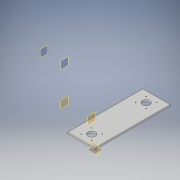
# Autodesk Inventor part: BT001_trajan20_21
Saved by Autodesk Inventor 2022.2 (Build 262287000, 287)
## iProperties
Company: HTBLA Kaindorf
RuleStatus: InUse
Created: 2022-06-05
Part Number: BT001_trajan20_21
Project: Zeichenmaschine_v2
Material: Generisch
Description: Gerüst
Document SubType Name: Modeling
Designer: trajan20
Density: 1 g/cm^3
Appearance: Vorgabe
Mass: 84.0087 g
Surface Area: 376.036 cm^2
Volume: 84.0087 cm^3
AfterDocNew0: iProperties-Editor_aufrufen
Author: jan
Keywords: 2021
Autodesk Inventor part; units mm, degrees
ref_plane "YZ Plane" through (0, 0, 0) normal (1, 0, 0) x (0, 1, 0)
ref_plane "XZ Plane" through (0, 0, 0) normal (0, 1, 0) x (-1, 0, 0)
ref_plane "XY Plane" through (0, 0, 0) normal (0, 0, 1) x (1, 0, 0)
derived "MS000_trajan20_21_Zeichenmaschine_Inventor_Masterskizze.ipt"
sketch "Skizze16" plane through (110, 40, -80) normal (1, 0, 0) x (0, 1, 0)
  line L0 (0, 0) -> (-80, 0)
  line L1 (-80, 0) -> (-80, -5)
  line L2 (-80, -5) -> (0, -5)
  line L3 (0, -5) -> (0, 0)
  point P0 (-40, 80)
sketch "Skizze17" plane through (110, 40, -85) normal (0, 0, -1) x (-1, 0, 0)
  line L0 (110, -322) -> (110, 182)
  line L1 (134, -40) -> (-34, -40)
  point P0 (110, -40)
  point P1 (30, -40)
  point P2 (14.5, -55.5)
  point P3 (45.5, -55.5)
  point P4 (14.5, -24.5)
  point P5 (45.5, -24.5)
extrude "Extrusion3" add sketch "Skizze16" against normal blind 110
sketch "Skizze5" plane through (110, -40, -85) normal (0, 0, -1) x (-1, 0, 0)
  point P0 (110, 40)
  point P1 (30, 40)
  point P2 (30, 40)
  constraints: 1 coincident
hole "Bohrung1" at (95.5, -15.5, -85) at (95.5, 15.5, -85) at (64.5, 15.5, -85) at (64.5, -15.5, -85) direction (0, 0, 1) diameter 2.459 end through all thread size "M3x0.5" class "6H" standard "ISO Metric profile"
hole "Bohrung2" at (80, 0, -85) direction (0, 0, 1) diameter 22 end through all
mirror "Spiegeln1" about plane through (0, 0, -82.5) normal (-1, 0, 0)
ref_plane "Arbeitsebene7" through (120, 40, 0) normal (0, 1, 0) x (-1, 0, 0)
ref_plane "Arbeitsebene8" through (120, -40, 0) normal (0, 1, 0) x (-1, 0, 0)
ref_plane "Arbeitsebene9" through (20, -200, 0) normal (0, -1, 0) x (1, 0, 0)
ref_plane "Arbeitsebene10" through (20, -140, 0) normal (0, -1, 0) x (1, 0, 0)
ref_plane "Arbeitsebene12" through (110, 40, -80) normal (1, 0, 0) x (0, 1, 0)
ref_plane "Arbeitsebene13" through (110, 40, -85) normal (0, 0, -1) x (-1, 0, 0)
equation "\"d5\" = 0.5 * Bas_Haupt_Länge"
equation "\"d14\" = SM_Scheibe_Durchmesser"
equation "\"Bas_Haupt_Länge\" = 220"
equation "\"SM_Scheibe_Durchmesser\" = 22"
